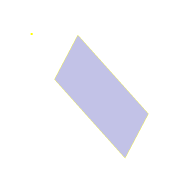
# Autodesk Inventor part: 07_OPENTRONS_Autofocus_objectivemount_v0
Saved by Autodesk Inventor 2019.4 (Build 234330000, 330)
## iProperties
Created: 2020-11-20
Part Number: 07_OPENTRONS_Autofocus_objectivemount_v0
Material: Generic
Document SubType Name: Modeling
Designer: diederichbenedict
Density: 1 g/cm^3
Appearance: Default
Author: diederichbenedict
Autodesk Inventor part; units mm, degrees
ref_plane "YZ Plane" through (0, 0, 0) normal (1, 0, 0) x (0, 1, 0)
ref_plane "XZ Plane" through (0, 0, 0) normal (0, 1, 0) x (-1, 0, 0)
ref_plane "XY Plane" through (0, 0, 0) normal (0, 0, 1) x (1, 0, 0)
ref_plane "Work Plane2" through (43.8996, -9.2473, 53.4016) normal (0, 0, 1) x (1, 0, 0)
sketch "Sketch2" plane through (43.8996, -9.2473, 53.4016) normal (0, 0, 1) x (1, 0, 0)
  circle A0 centre (-10.125, 0) radius 12.15 construction
  arc A1 (-14.1278, 12) -> (-6.1222, 12) centre (-10.125, 0) ccw
  circle A2 centre (-10.125, 0) radius 15
  line L0 (-14.1278, 12) -> (-6.1222, 12)
  point P0 (-43.8996, 9.2473)
  point P1 (-14.1278, 12)
  point P2 (-6.1222, 12)
  dimension "d0" = 0.5
  dimension "d1" = 30
  dimension "d2" = 12
  constraints: 3 coincident, 2 centre point, 2 end point, 2 point on circle, 1 horizontal
  measures "d0" radial gap between concentric circles of A0 A1
  measures "d1" diameter of A2
  measures "d2" distance from line of A0.centre L0
extrude "Extrusion1" add sketch "Sketch2" against normal blind 6
pattern_circular "Circular Pattern1" count 3 over 360 about axis through (33.7746, -9.2473, 53.4016) along (0, 0, -1) of "Extrusion1"
body "Solid1"
